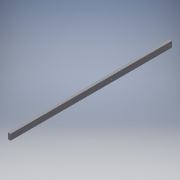
# Autodesk Inventor part: Trebuchet Arm
Saved by Autodesk Inventor 2019 (Build 230136000, 136)
## iProperties
Created: 2019-07-10
Part Number: Trebuchet Arm
Material: Generic
Document SubType Name: Modeling
Designer: AlphaGoldOmegaSilver
Density: 1 g/cm^3
Appearance: Default
Mass: 8249.43 g
Surface Area: 6286.61 cm^2
Volume: 8249.43 cm^3
Author: AlphaGoldOmegaSilver
Autodesk Inventor part; units mm, degrees
ref_plane "YZ Plane" through (0, 0, 0) normal (1, 0, 0) x (0, 1, 0)
ref_plane "XZ Plane" through (0, 0, 0) normal (0, 1, 0) x (-1, 0, 0)
ref_plane "XY Plane" through (0, 0, 0) normal (0, 0, 1) x (1, 0, 0)
sketch "Sketch1" plane through (0, 0, 0) normal (1, 0, 0) x (0, 1, 0)
  line L0 (44.45, 1219.2) -> (-44.45, 1219.2)
  line L1 (-44.45, 1219.2) -> (-44.45, -1219.2)
  line L2 (-44.45, -1219.2) -> (44.45, -1219.2)
  line L3 (44.45, -1219.2) -> (44.45, 1219.2)
  line L4 (44.45, 1219.2) -> (-44.45, -1219.2) construction
  line L5 (-44.45, 1219.2) -> (44.45, -1219.2) construction
  line L6 (44.45, -1219.2) -> (-44.45, -1219.2) construction
  line L7 (-44.45, -1219.2) -> (-44.45, -1181.1) construction
  line L8 (-44.45, -1181.1) -> (44.45, -1181.1) construction
  line L9 (44.45, -1181.1) -> (44.45, -1219.2) construction
  circle A0 centre (0, -1181.1) radius 6.35
  point P0 (0, 0)
  dimension "d0" = 88.9
  dimension "d1" = 2438.4
  dimension "d2" = 88.9
  dimension "d3" = 38.1
  dimension "d4" = 12.7
  constraints: 20 end point, 4 parallel, 3 midpoint, 2 horizontal, 2 perpendicular, 1 centre point
  measures "d0" distance of L2.end L1.end
  measures "d1" distance of L1.end L0.end
  measures "d2" distance of L7.end L8.end
  measures "d3" distance of L6.end L7.end
  measures "d4" diameter of A0
extrude "Extrusion1" add sketch "Sketch1" along normal blind 38.1
sketch "Sketch2" plane through (38.1, 0, 0) normal (1, 0, 0) x (0, 0, -1)
  circle A0 centre (1181.1, 0) radius 6.35 projected
  line L0 (1181.1, 0) -> (304.8, 0) construction
  circle A1 centre (304.8, 0) radius 6.35
  point P0 (0, 0)
  dimension "d7" = 876.3
  dimension "d8" = 12.7
  constraints: 2 end point, 1 centre point, 1 coincident, 1 horizontal
  measures "d7" distance of L0.start L0.end
  measures "d8" diameter of A1
extrude "Extrusion2" cut sketch "Sketch2" against normal blind 38.1 contours A1
body "Solid1"
